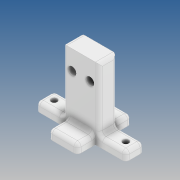
# Autodesk Inventor part: 2114_Nut Plate Support_V1
Saved by Autodesk Inventor 2020 (Build 240168000, 168)
## iProperties
Created: 2019-11-08
Part Number: 2114_Nut Plate Support_V1
Material: ABS Plastic
Document SubType Name: Modeling
Designer: RFLab
Density: 1.06 g/cm^3
Appearance: Smooth - White
Author: RFLab
Autodesk Inventor part; units mm, degrees
ref_plane "YZ Plane" through (0, 0, 0) normal (1, 0, 0) x (0, 1, 0)
ref_plane "XZ Plane" through (0, 0, 0) normal (0, 1, 0) x (-1, 0, 0)
ref_plane "XY Plane" through (0, 0, 0) normal (0, 0, 1) x (1, 0, 0)
sketch "Sketch1" plane through (0, 0, 0) normal (0, 0, 1) x (1, 0, 0)
  line L0 (-10, 20) -> (10, 20)
  line L1 (10, 20) -> (10, -20)
  line L2 (10, -20) -> (-10, -20)
  line L3 (-10, -20) -> (-10, 20)
  point P0 (0, 0)
  dimension "d0" = 20
  dimension "d1" = 10
  dimension "d2" = 20
  dimension "d3" = 40
  constraints: 8 end point, 2 parallel, 1 horizontal, 1 perpendicular
  measures "d0" distance from line of point (0, 0) L0
  measures "d1" distance from line of L3 point (0, 0)
  measures "d2" distance of L1.end L2.end
  measures "d3" distance of L0.end L1.end
extrude "Extrusion1" add sketch "Sketch1" along normal blind 10
sketch "Sketch2" plane through (10, -20, 0) normal (1, 0, 0) x (0, 0, -1)
  line L0 (-10, 0) -> (-10, 40) projected
  line L1 (-10, 0) -> (0, 0)
  line L2 (0, 0) -> (0, 5)
  line L3 (0, 5) -> (-10, 5)
  line L4 (-10, 5) -> (-10, 0)
  line L5 (0, 0) -> (0, 40) projected
  point P0 (0, 20)
  dimension "d6" = 5
  constraints: 8 end point, 2 parallel, 1 horizontal, 1 perpendicular, 1 point on line
  measures "d6" distance of L2.end L1.end
extrude "Extrusion2" add sketch "Sketch2" along normal blind 15
sketch "Sketch3" plane through (-10, -20, 0) normal (-1, 0, 0) x (0, 0, 1)
  line L0 (0, 0) -> (10, 0) projected
  line L1 (10, 40) -> (10, 0) projected
  line L2 (0, 0) -> (10, 0)
  line L3 (10, 0) -> (10, 5)
  line L4 (10, 5) -> (0, 5)
  line L5 (0, 5) -> (0, 0)
  point P0 (0, 20)
  dimension "d9" = 5
  constraints: 8 end point, 2 parallel, 1 horizontal, 1 perpendicular, 1 point on line
  measures "d9" distance of L0.end L3.end
extrude "Extrusion3" add sketch "Sketch3" along normal blind 15
sketch "Sketch4" plane through (0, 0, 10) normal (0, 0, 1) x (1, 0, 0)
  circle A0 centre (-5, 9.15) radius 2.3
  line L0 (25, -20) -> (-25, -20) projected
  line L1 (-10, 20) -> (-10, -15) projected
  circle A1 centre (5, 9.15) radius 2.3
  line L2 (10, -15) -> (10, 20) projected
  point P0 (0, 0)
  dimension "d12" = 29.15
  dimension "d13" = 4.6
  dimension "d36" = 5
  dimension "d37" = 5
  dimension "d38" = 29.15
  constraints: 2 centre point, 1 equal radius
  measures "d12" distance from line of L0 A0.centre
  measures "d13" diameter of A0
  measures "d36" distance from line of L1 A0.centre
  measures "d37" distance from line of L2 A1.centre
  measures "d38" distance from line of L0 A1.centre
extrude "Extrusion4" cut sketch "Sketch4" against normal through all
sketch "Sketch5" plane through (10, -15, 10) normal (0, 1, 0) x (1, 0, 0)
  circle A0 centre (-11.0524, 5.4355) radius 1.65
  circle A1 centre (-30, 5) radius 1.65
  line L0 (-35, 0) -> (-35, 10) projected
  line L1 (-20, 10) -> (-35, 10) projected
  circle A2 centre (10, 5) radius 1.65
  line L2 (15, 10) -> (15, 0) projected
  line L3 (0, 10) -> (15, 10) projected
  point P0 (-10, 10)
  dimension "d16" = 3.3
  dimension "d17" = 5
  dimension "d18" = 5
  dimension "d19" = 5
  dimension "d20" = 5
  constraints: 3 centre point, 2 equal radius
  measures "d16" diameter of A1
  measures "d17" distance from line of L0 A1.centre
  measures "d18" distance from line of L1 A1.centre
  measures "d19" distance from line of L2 A2.centre
  measures "d20" distance from line of L3 A2.centre
extrude "Extrusion5" cut sketch "Sketch5" against normal through all contours A1 | A2
fillet "Fillet1" radius 2 6 edges at (-25, -17.5, 0) (-25, -17.5, 10) (25, -17.5, 0) (25, -17.5, 10) (10, -15, 5) (-10, -15, 5)
fillet "Fillet2" radius 2 20 edges at (10, 20, 5) (-10, 20, 5) (-10.5858, -14.4142, 0) (-17.5, -15, 0) (-24.4142, -15, 0.5858) (-25, -15, 5) (-24.4142, -15, 9.4142) (-17.5, -15, 10) (-10.5858, -14.4142, 10) (-10, 3.5, 10) (-10, 3.5, 0) (10.5858, -14.4142, 0) (17.5, -15, 0) (24.4142, -15, 0.5858) (25, -15, 5) (24.4142, -15, 9.4142) (17.5, -15, 10) (10.5858, -14.4142, 10) (10, 3.5, 10) (10, 3.5, 0)
sketch "Sketch6" plane through (0, 0, 0) normal (0, 0, -1) x (-1, 0, 0)
  line L0 (-23, -20) -> (23, -20) projected
  line L1 (-8, -20) -> (8, -20)
  line L2 (8, -20) -> (8, -15)
  line L3 (8, -15) -> (-8, -15)
  line L4 (-8, -15) -> (-8, -20)
  point P0 (0, 0)
  point P1 (8, -20)
  dimension "d25" = 15
  dimension "d26" = 15
  dimension "d29" = 5
  constraints: 8 end point, 2 parallel, 1 horizontal, 1 perpendicular, 1 point on line
  measures "d25" distance of L0.start L1.start
  measures "d26" distance of L0.end L1.end
  measures "d29" distance of L3.end L1.start
extrude "Extrusion6" add sketch "Sketch6" along normal blind 10
sketch "Sketch7" plane through (0, 0, 10) normal (0, 0, 1) x (1, 0, 0)
  line L0 (23, -20) -> (-23, -20) projected
  line L1 (-8, -20) -> (8, -20)
  line L2 (8, -20) -> (8, -15)
  line L3 (8, -15) -> (-8, -15)
  line L4 (-8, -15) -> (-8, -20)
  point P0 (0, 0)
  point P1 (8, -20)
  dimension "d30" = 15
  dimension "d31" = 15
  dimension "d32" = 5
  constraints: 8 end point, 2 parallel, 1 horizontal, 1 perpendicular, 1 point on line
  measures "d30" distance of L1.start L0.end
  measures "d31" distance of L0.start L1.end
  measures "d32" distance of L1.end L2.end
extrude "Extrusion7" add sketch "Sketch7" along normal blind 10
fillet "Fillet3" radius 2 12 edges at (8, -15, 15) (0, -15, 10) (-8, -15, 15) (0, -15, 20) (8, -17.5, 20) (-8, -17.5, 20) (0, -15, 0) (8, -15, -5) (8, -17.5, -10) (0, -15, -10) (-8, -15, -5) (-8, -17.5, -10)
equation "\"d0\" = 0.5 * d3"
equation "\"d1\" = 0.5 * d2"
equation "\"d37\" = d36"
equation "\"d38\" = d12"
equation "\"d26\" = d25"
equation "\"d31\" = d30"
body "Solid1"
